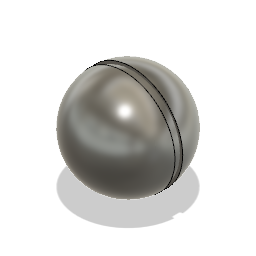
pokeball v2 (Autodesk Fusion 360 design; units mm, degrees)
Autodesk Fusion 360 part; units mm, degrees
note: some values were not read from the file. Set by a fixed rule: which sketch regions a step uses.
sketch "Sketch4" plane through (0, 0, 0) normal (0, 1, 0) x (1, 0, 0)
  circle A0 centre (0, 0) radius 5
  line L0 (0, 7) -> (0, -7.4768)
  line L1 (-8, 0) -> (8, 0)
  line L2 (-11.6654, 0.375) -> (11.6654, 0.375)
  line L3 (11.6654, 0.375) -> (11.6654, -0.375)
  line L4 (11.6654, -0.375) -> (-11.6654, -0.375)
  line L5 (-11.6654, -0.375) -> (-11.6654, 0.375)
  line L6 (-11.6654, 0.375) -> (11.6654, -0.375) construction
  line L7 (11.6654, 0.375) -> (-11.6654, -0.375) construction
  dimension "d4" = 10
  dimension "d5" = 0.75
  constraint coincident A0.centre origin
  constraint vertical L0
  constraint horizontal L1
  constraint horizontal L2
  constraint perpendicular L2 L3
  constraint parallel L2 L4
  constraint parallel L3 L5
  constraint coincident L6 A0.centre
  constraint coincident L7 A0.centre
  measures "d4" diameter of A0
  measures "d5" distance of L2.end L3.end
revolve "Revolve1" add sketch "Sketch4" angle 360 about axis through (0, 0, -7) along (0, 0, 1) contours A0 L0 L4 | A0 L0 L2 picked at (3.2868, -0.6213) picked at (-3.2868, 0.6213) makes body 1 at (2.4503, 4.2441, -0.9919) makes body 2 at (2.4503, -4.2441, 0.9919)
sketch "Sketch5" plane through (0, 0, 0) normal (0, 1, 0) x (1, 0, 0)
  circle A0 centre (0, 0) radius 4.75
  line L0 (0, 7) -> (0, -7)
  dimension "d7" = 9.5
  constraint coincident A0.centre origin
  constraint vertical L0
  measures "d7" diameter of A0
revolve "Revolve2" add sketch "Sketch5" angle 360 about axis through (0, 0, -7) along (0, 0, 1) separate body contours A0 L0 picked at (1.4219, 1.0207) makes body 3
